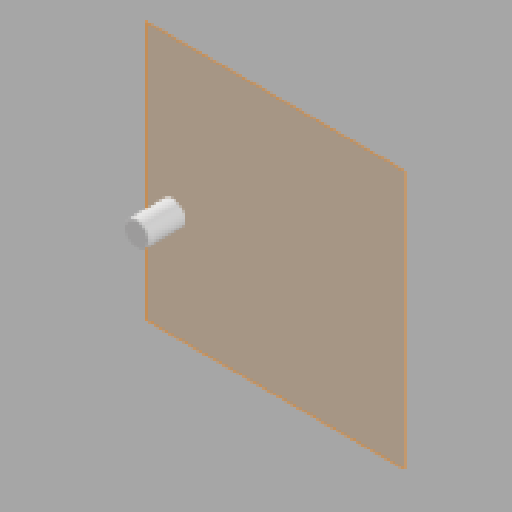
# Autodesk Inventor part: Spacers
Saved by Autodesk Inventor 2027 (Build 310192060, 192F)
## iProperties
Created: 2026-06-26
Part Number: Spacers
Material: Generic
Document SubType Name: Modeling
Designer: opore
Density: 1 g/cm^3
Appearance: Default
Author: opore
Autodesk Inventor part; units mm, degrees
ref_plane "YZ Plane" through (0, 0, 0) normal (1, 0, 0) x (0, 1, 0)
ref_plane "XZ Plane" through (0, 0, 0) normal (0, 1, 0) x (-1, 0, 0)
ref_plane "XY Plane" through (0, 0, 0) normal (0, 0, 1) x (1, 0, 0)
ref_plane "Work Plane1" through (0, 0, 0) normal (0, 0, 1) x (1, 0, 0)
sketch "Sketch1" plane through (0, 0, 0) normal (0, 0, 1) x (1, 0, 0)
  circle A0 centre (-53.7689, -11.7651) radius 3.2332 projected
  circle A1 centre (-53.7689, -11.7651) radius 4.05
  circle A2 centre (-53.7689, -11.7651) radius 6.5
  point P0 (0, 0)
  point P1 (-52.2586, -9.305)
  dimension "d0" = 8.1
  dimension "d1" = 13
  constraints: 2 centre point, 2 coincident, 1 other
  measures "d0" diameter of A1
  measures "d1" diameter of A2
extrude "Extrusion1" add sketch "Sketch1" along normal blind 20 contours A0 | A1 | A2
chamfer "Chamfer1" distance 0.5 angle 45 2 edges at (-60.2689, -11.7651, 0) (-60.2689, -11.7651, 20)
sketch "Sketch2" plane through (-53.7689, -11.7651, 20) normal (0, 0, 1) x (1, 0, 0)
  circle A0 centre (0, 0) radius 4.05
  point P0 (53.7689, 11.7651)
  dimension "d7" = 8.1
  constraints: 1 centre point
  measures "d7" diameter of A0
extrude "Extrusion2" cut sketch "Sketch2" against normal blind 20
body "Solid1"
